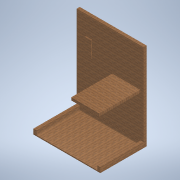
# Autodesk Inventor part: Base model
Saved by Autodesk Inventor 2021 (Build 250183000, 183)
## iProperties
Created: 2021-06-29
Part Number: Base model
Material: Wood (Maple)
Document SubType Name: Modeling
Designer: HP
Density: 0.67 g/cm^3
Appearance: White Ash - Java
Author: HP
Autodesk Inventor part; units mm, degrees
ref_plane "YZ Plane" through (0, 0, 0) normal (1, 0, 0) x (0, 1, 0)
ref_plane "XZ Plane" through (0, 0, 0) normal (0, 1, 0) x (-1, 0, 0)
ref_plane "XY Plane" through (0, 0, 0) normal (0, 0, 1) x (1, 0, 0)
sketch "Sketch1" plane through (0, 0, 0) normal (0, 1, 0) x (-1, 0, 0)
  line L0 (6489.7905, 4493.7678) -> (-10.2095, 4493.7678)
  line L1 (-10.2095, 4493.7678) -> (-10.2095, -6.2322)
  line L2 (-10.2095, -6.2322) -> (6489.7905, -6.2322)
  line L3 (6489.7905, -6.2322) -> (6489.7905, 4493.7678)
  point P0 (0, 0)
  dimension "d0" = 6500
  dimension "d1" = 4500
  constraints: 8 end point, 2 parallel, 1 horizontal, 1 perpendicular
  measures "d0" distance of L2.end L1.end
  measures "d1" distance between parallel lines of L0 L2
extrude "Extrusion1" add sketch "Sketch1" along normal blind 500
sketch "Sketch6" plane through (0, 500, 0) normal (0, 1, 0) x (1, 0, 0)
  line L0 (-6189.7905, -293.7678) -> (-289.7905, -293.7678)
  line L1 (-289.7905, -293.7678) -> (-289.7905, -4193.7678)
  line L2 (-289.7905, -4193.7678) -> (-6189.7905, -4193.7678)
  line L3 (-6189.7905, -4193.7678) -> (-6189.7905, -293.7678)
  line L4 (10.2095, 6.2322) -> (-6489.7905, 6.2322) projected
  line L5 (-6489.7905, -4493.7678) -> (10.2095, -4493.7678) projected
  line L6 (-6489.7905, 6.2322) -> (-6489.7905, -4493.7678) projected
  line L7 (10.2095, -4493.7678) -> (10.2095, 6.2322) projected
  point P0 (0, 0)
  dimension "d22" = 300
  dimension "d23" = 300
  dimension "d24" = 300
  dimension "d25" = 300
  constraints: 8 end point, 2 parallel, 1 horizontal, 1 perpendicular
  measures "d22" distance between parallel lines of L0 L4
  measures "d23" distance between parallel lines of L2 L5
  measures "d24" distance between parallel lines of L3 L6
  measures "d25" distance between parallel lines of L1 L7
extrude "Extrusion5" cut sketch "Sketch6" against normal blind 400 contours L0 L1 L2 L3
sketch "Sketch7" plane through (0, 500, 0) normal (0, 1, 0) x (1, 0, 0)
  line L0 (-6489.7905, 6.2322) -> (-6489.7905, -4493.7678) projected
  line L1 (10.2095, -4493.7678) -> (10.2095, 6.2322) projected
  line L2 (-6489.7905, 6.2322) -> (10.2095, 6.2322)
  line L3 (10.2095, 6.2322) -> (10.2095, -284.9992)
  line L4 (10.2095, -284.9992) -> (-6489.7905, -284.9992)
  line L5 (-6489.7905, -284.9992) -> (-6489.7905, 6.2322)
  point P0 (0, 0)
  constraints: 8 end point, 2 parallel, 1 horizontal, 1 perpendicular, 1 point on line
extrude "Extrusion6" add sketch "Sketch7" along normal blind 8000
sketch "Sketch8" plane through (-6489.7905, 0, 4493.7678) normal (0, 0, 1) x (1, 0, 0)
  line L0 (6200, 500) -> (300, 500) projected
  line L1 (300, 500) -> (6200, 500)
  line L2 (6200, 500) -> (6200, 100)
  line L3 (6200, 100) -> (300, 100)
  line L4 (300, 100) -> (300, 500)
  line L5 (6500, 0) -> (6500, 500) projected
  line L6 (0, 0) -> (6500, 0) projected
  point P0 (6489.7905, 0)
  dimension "d30" = 300
  dimension "d31" = 100
  constraints: 8 end point, 2 parallel, 1 horizontal, 1 perpendicular
  measures "d30" distance between parallel lines of L2 L5
  measures "d31" distance between parallel lines of L3 L6
extrude "Extrusion7" cut sketch "Sketch8" against normal blind 300
sketch "Sketch9" plane through (-6489.7905, 500, 284.9992) normal (0, 0, 1) x (1, 0, 0)
  line L0 (3460.9411, 4259.6208) -> (6185.9849, 4259.6208)
  line L1 (6185.9849, 4259.6208) -> (6185.9849, 4001.8464)
  line L2 (6185.9849, 4001.8464) -> (3460.9411, 4001.8464)
  line L3 (3460.9411, 4001.8464) -> (3460.9411, 4259.6208)
  line L4 (165.1111, 1221.565) -> (2853.33, 1221.565)
  line L5 (2853.33, 1221.565) -> (2853.33, 908.5532)
  line L6 (2853.33, 908.5532) -> (165.1111, 908.5532)
  line L7 (165.1111, 908.5532) -> (165.1111, 1221.565)
  point P0 (6489.7905, -500)
  constraints: 16 end point, 4 parallel, 2 horizontal, 2 perpendicular
extrude "Extrusion8" add sketch "Sketch9" along normal blind 4000 contours L0 L1 L2 L3
sketch "Sketch11" plane through (-6489.7905, 500, 284.9992) normal (0, 0, 1) x (1, 0, 0)
  line L0 (901.7669, 6134.2214) -> (1499.5941, 6134.2214)
  line L1 (1499.5941, 6134.2214) -> (1499.5941, 4540.0155)
  line L2 (1499.5941, 4540.0155) -> (901.7669, 4540.0155)
  line L3 (901.7669, 4540.0155) -> (901.7669, 6134.2214)
  point P0 (6489.7905, -500)
  constraints: 8 end point, 2 parallel, 1 horizontal, 1 perpendicular
extrude "Extrusion10" add sketch "Sketch11" along normal blind 120
body "Solid1"
